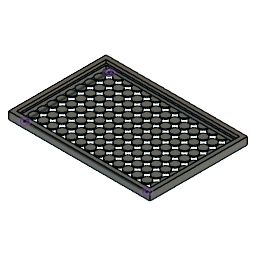
Darkfield 96 2.0 (Autodesk Fusion 360 design; units mm, degrees)
Autodesk Fusion 360 part; units mm, degrees
note: some values were not read from the file. Chosen so that the rebuilt part matches the saved one: which bodies a step acts on; which face or edge a step refers to.
sketch "Sketch1" plane through (0, 0, 0) normal (0, 0, 1) x (1, 0, 0)
  line L0 (0, 0) -> (127.6, 0)
  line L1 (127.6, 0) -> (127.6, 85.5)
  line L2 (127.6, 85.5) -> (0, 85.5)
  line L3 (0, 85.5) -> (0, 0)
  dimension "d1" = 127.6
  dimension "d2" = 85.5
  constraint horizontal L0
  constraint vertical L1
  constraint horizontal L2
  constraint vertical L3
  constraint coincident L0.start L3.end
  measures "d1" distance of L0.start L0.end
  measures "d2" distance of L0.start L2.end
ref_plane "WorkPlane1" through (0, 0, 0) normal (0, -1, 0) x (1, 0, 0)
sketch "Sketch2" plane through (0, 0, 0) normal (0, -1, 0) x (1, 0, 0)
  line L0 (0, 0) -> (0, 3)
  line L1 (0, 3) -> (-3.9, 3)
  line L2 (-3.9, 3) -> (-3.9, -4)
  line L3 (-3.9, -4) -> (1.6, -4)
  line L4 (1.6, -4) -> (1.6, 0)
  line L5 (0, 0) -> (1.6, 0)
  line L6 (-3.9, -3) -> (1.6, -3)
  line L7 (0, 0) -> (127.6, 0)
  dimension "d4" = 3
  dimension "d6" = 1
  dimension "d7" = 3
  dimension "d8" = 3.9
  dimension "d9" = 5.5
  constraint coincident L0.start L5.start
  constraint vertical L0
  constraint perpendicular L0 L1
  constraint perpendicular L1 L2
  constraint perpendicular L2 L3
  constraint perpendicular L1 L4
  constraint perpendicular L4 L5
  constraint coincident L2 L6.start
  constraint coincident L4 L6.end
  constraint perpendicular L4 L6
  measures "d4" distance of L0.start L0.end
  measures "d6" distance of L3 L6
  measures "d7" distance of L6 L7
  measures "d8" distance of L0 L2
  measures "d9" distance of L2 L4
sweep "Sweep1" add profiles "Sketch2" path "Sketch1" along L3 L0 L1 L2 section 1 makes body 1
sketch "Sketch3" plane through (0, 0, -4) normal (0, 0, 1) x (-1, 0, 0)
  line L0 (0, 0) -> (-127.6, 0)
  line L1 (-127.6, 0) -> (-127.6, -85.5)
  line L2 (-127.6, -85.5) -> (0, -85.5)
  line L3 (0, -85.5) -> (0, 0)
  line L4 (-126, -1.6) -> (-1.6, -1.6)
  line L5 (-1.6, -1.6) -> (-1.6, -83.9)
  line L6 (-1.6, -83.9) -> (-126, -83.9)
  line L7 (-126, -83.9) -> (-126, -1.6)
  circle A0 centre (-14.2, -11.3) radius 4
  line L8 (3.9, 3.9) -> (3.9, -89.4)
  line L9 (3.9, -89.4) -> (-131.5, -89.4)
  line L10 (-131.5, -89.4) -> (-131.5, 3.9)
  line L11 (-131.5, 3.9) -> (3.9, 3.9)
  line L12 (-126, -1.6) -> (-126, -83.9)
  line L13 (-126, -83.9) -> (-1.6, -83.9)
  line L14 (-1.6, -83.9) -> (-1.6, -1.6)
  line L15 (-1.6, -1.6) -> (-126, -1.6)
  dimension "d16" = 14.2
  dimension "d17" = 11.3
  dimension "d18" = 8
  measures "d16" distance of L3 A0.centre
  measures "d17" distance of L0 A0.centre
  measures "d18" diameter of A0
extrude "Extrude1" add sketch "Sketch3" along normal blind 1 separate body contours A0 makes body 2
pattern_linear "R-Pattern1" count 12 spacing 9.0182 along (1, 0, 0) count 8 spacing 8.9857 along (0, 1, 0) of bodies 2 makes body 3 at (24.2224, 11.9082, -4) makes body 4 at (34.8289, 11.8917, -4) makes body 5 at (42.2588, 11.9082, -4) makes body 6 at (52.8653, 11.8917, -4) makes body 7 at (61.8834, 11.8917, -4) makes body 8 at (70.9016, 11.8917, -4) makes body 9 at (79.9198, 11.8917, -4) makes body 10 at (88.938, 11.8917, -4) makes body 11 at (97.9562, 11.8917, -4) makes body 12 at (106.9744, 11.8917, -4) makes body 13 at (115.9925, 11.8917, -4) makes body 14 at (13.0255, 19.4085, -4) makes body 15 at (22.1898, 21.3579, -4) makes body 16 at (34.0244, 19.6188, -4) makes body 17 at (40.2262, 21.3579, -4) makes body 18 at (52.0608, 19.6188, -4) makes body 19 at (61.079, 19.6188, -4) makes body 20 at (70.0971, 19.6188, -4) makes body 21 at (79.1153, 19.6188, -4) makes body 22 at (88.1335, 19.6188, -4) makes body 23 at (97.1517, 19.6188, -4) makes body 24 at (106.1699, 19.6188, -4) makes body 25 at (115.1881, 19.6188, -4) makes body 26 at (15.3745, 28.3348, -4) makes body 27 at (24.6188, 29.8499, -4) makes body 28 at (34.2215, 28.6342, -4) makes body 29 at (42.6551, 29.8499, -4) makes body 30 at (52.2578, 28.6342, -4) makes body 31 at (61.276, 28.6342, -4) makes body 32 at (70.2942, 28.6342, -4) makes body 33 at (79.3124, 28.6342, -4) makes body 34 at (88.3306, 28.6342, -4) makes body 35 at (97.3487, 28.6342, -4) makes body 36 at (106.3669, 28.6342, -4) makes body 37 at (115.3851, 28.6342, -4) makes body 38 at (13.5921, 37.6786, -4) makes body 39 at (24.4195, 38.8357, -4) makes body 40 at (33.9068, 38.6204, -4) makes body 41 at (40.4232, 39.2996, -4) makes body 42 at (51.9432, 38.6204, -4) makes body 43 at (60.9613, 38.6204, -4) makes body 44 at (69.9795, 38.6204, -4) makes body 45 at (78.9977, 38.6204, -4) makes body 46 at (88.0159, 38.6204, -4) makes body 47 at (97.0341, 38.6204, -4) makes body 48 at (106.0522, 38.6204, -4) makes body 49 at (115.0704, 38.6204, -4) makes body 50 at (13.5921, 46.6643, -4) makes body 51 at (24.4195, 47.8214, -4) makes body 52 at (33.9068, 47.6062, -4) makes body 53 at (40.4232, 48.2853, -4) makes body 54 at (51.9432, 47.6062, -4) makes body 55 at (60.9613, 47.6062, -4) makes body 56 at (69.9795, 47.6062, -4) makes body 57 at (78.9977, 47.6062, -4) makes body 58 at (88.0159, 47.6062, -4) makes body 59 at (97.0341, 47.6062, -4) makes body 60 at (106.0522, 47.6062, -4) makes body 61 at (115.0704, 47.6062, -4) makes body 62 at (13.5921, 55.6501, -4) makes body 63 at (24.4195, 56.8071, -4) makes body 64 at (33.9068, 56.5919, -4) makes body 65 at (40.4232, 57.271, -4) makes body 66 at (51.9432, 56.5919, -4) makes body 67 at (60.9613, 56.5919, -4) makes body 68 at (69.9795, 56.5919, -4) makes body 69 at (78.9977, 56.5919, -4) makes body 70 at (88.0159, 56.5919, -4) makes body 71 at (97.0341, 56.5919, -4) makes body 72 at (106.0522, 56.5919, -4) makes body 73 at (115.0704, 56.5919, -4) makes body 74 at (16.3023, 65.3543, -4) makes body 75 at (24.8158, 65.8225, -4) makes body 76 at (34.031, 64.6358, -4) makes body 77 at (42.8522, 65.8225, -4) makes body 78 at (52.0674, 64.6358, -4) makes body 79 at (61.0856, 64.6358, -4) makes body 80 at (70.1038, 64.6358, -4) makes body 81 at (79.122, 64.6358, -4) makes body 82 at (88.1401, 64.6358, -4) makes body 83 at (97.1583, 64.6358, -4) makes body 84 at (106.1765, 64.6358, -4) makes body 85 at (115.1947, 64.6358, -4) makes body 86 at (16.3023, 74.34, -4) makes body 87 at (24.8158, 74.8082, -4) makes body 88 at (34.031, 73.6215, -4) makes body 89 at (42.8522, 74.8082, -4) makes body 90 at (52.0674, 73.6215, -4) makes body 91 at (61.0856, 73.6215, -4) makes body 92 at (70.1038, 73.6215, -4) makes body 93 at (79.122, 73.6215, -4) makes body 94 at (88.1401, 73.6215, -4) makes body 95 at (97.1583, 73.6215, -4) makes body 96 at (106.1765, 73.6215, -4) makes body 97 at (115.1947, 73.6215, -4)
sketch "Sketch4" plane through (0, 0, -3) normal (0, 0, 1) x (-1, 0, 0)
  circle A0 centre (-14.2, -74.2) radius 4
  circle A1 centre (-14.2, -65.2143) radius 4
  circle A2 centre (-23.2182, -74.2) radius 4
  dimension "d25" = 8.9857
  dimension "d26" = 9.0182
  measures "d25" distance of A0.centre A1.centre
  measures "d26" distance of A0.centre A2.centre
pattern_linear "R-Pattern2" count 2 spacing 8.9857 along (0, 1, 0) of bodies 86 87 88 89 96 97 90 95 92 91 93 94 makes body 98 at (16.3023, 83.3257, -4) makes body 99 at (24.8158, 83.7939, -4) makes body 100 at (34.031, 82.6072, -4) makes body 101 at (42.8522, 83.7939, -4) makes body 102 at (52.0674, 82.6072, -4) makes body 103 at (61.0856, 82.6072, -4) makes body 104 at (70.1038, 82.6072, -4) makes body 105 at (79.122, 82.6072, -4) makes body 106 at (88.1401, 82.6072, -4) makes body 107 at (97.1583, 82.6072, -4) makes body 108 at (106.1765, 82.6072, -4) makes body 109 at (115.1947, 82.6072, -4)
pattern_linear "R-Pattern3" count 2 spacing 9.0182 along (-1, 0, 0) of bodies 2 14 26 38 50 62 74 86 98 makes body 110 at (6.8966, 11.469, -4) makes body 111 at (4.0074, 19.4085, -4) makes body 112 at (6.3563, 28.3348, -4) makes body 113 at (4.5739, 37.6786, -4) makes body 114 at (4.5739, 46.6643, -4) makes body 115 at (4.5739, 55.6501, -4) makes body 116 at (7.2841, 65.3543, -4) makes body 117 at (7.2841, 74.34, -4) makes body 118 at (7.2841, 83.3257, -4)
ref_plane "WorkPlane2" through (63.8, 42.75, -0.5) normal (-1, 0, 0) x (0, 0, -1)
ref_plane "WorkPlane3" through (63.8, 42.75, -0.5) normal (0, -1, 0) x (0, 0, -1)
ref_plane "WorkPlane4" through (-3.9, -3.9, -4) normal (0.567406, -0.823438, 0) x (0.823438, 0.567406, 0)
mirror "Mirror1" about plane through (63.8, 42.75, -0.5) normal (0, -1, 0) of bodies 105 106 108 109 98 99 100 102 104 101 103 118 107 makes body 119 at (15.9148, 2.1453, -4) makes body 120 at (24.2224, 1.7061, -4) makes body 121 at (34.8289, 1.7226, -4) makes body 122 at (42.2588, 1.7061, -4) makes body 123 at (52.8653, 1.7226, -4) makes body 124 at (61.8834, 1.7226, -4) makes body 125 at (70.9016, 1.7226, -4) makes body 126 at (79.9198, 1.7226, -4) makes body 127 at (88.938, 1.7226, -4) makes body 128 at (97.9562, 1.7226, -4) makes body 129 at (106.9744, 1.7226, -4) makes body 130 at (115.9925, 1.7226, -4) makes body 131 at (6.8966, 2.1453, -4)
mirror "Mirror2" about plane through (63.8, 42.75, -0.5) normal (-1, 0, 0) of bodies 131 110 111 112 113 115 114 116 117 118 makes body 132 at (119.8256, 11.8917, -4) makes body 133 at (120.6301, 19.6188, -4) makes body 134 at (120.4331, 28.6342, -4) makes body 135 at (120.7478, 38.6204, -4) makes body 136 at (120.7478, 47.6062, -4) makes body 137 at (120.7478, 56.5919, -4) makes body 138 at (120.6235, 64.6358, -4) makes body 139 at (120.6235, 73.6215, -4) makes body 140 at (120.6235, 82.6072, -4) makes body 141 at (119.8256, 1.7226, -4)
sketch "Sketch5" plane through (0, 0, -4) normal (0, 0, -1) x (1, 0, 0)
  line L0 (-3.9, 3.9) -> (-3.9, -89.4)
  line L1 (-3.9, -89.4) -> (131.5, -89.4)
  line L2 (131.5, -89.4) -> (131.5, 3.9)
  line L3 (131.5, 3.9) -> (-3.9, 3.9)
  line L4 (126, -1.6) -> (126, -83.9)
  line L5 (126, -83.9) -> (1.6, -83.9)
  line L6 (1.6, -83.9) -> (1.6, -1.6)
  line L7 (1.6, -1.6) -> (126, -1.6)
  circle A0 centre (5.1818, -2.3143) radius 4
  circle A1 centre (5.1818, -83.1857) radius 4
  circle A2 centre (122.4182, -2.3143) radius 4
  line L8 (5.1818, -1.8143) -> (122.4182, -1.8143)
  line L9 (122.4182, -1.8143) -> (122.4182, -2.8143)
  line L10 (122.4182, -2.8143) -> (5.1818, -2.8143)
  line L11 (5.1818, -2.8143) -> (5.1818, -1.8143)
  line L12 (4.6818, -2.3143) -> (5.6818, -2.3143)
  line L13 (5.6818, -2.3143) -> (5.6818, -83.1857)
  line L14 (5.6818, -83.1857) -> (4.6818, -83.1857)
  line L15 (4.6818, -83.1857) -> (4.6818, -2.3143)
  dimension "d39" = 1
  dimension "d40" = 1
  dimension "d41" = 80.8714
  dimension "d42" = 117.2364
  constraint horizontal L8
  constraint vertical L9
  constraint horizontal L10
  constraint vertical L11
  constraint midpoint A0.centre L11
  constraint horizontal L12
  constraint vertical L13
  constraint horizontal L14
  constraint vertical L15
  constraint midpoint A1.centre L14
  constraint midpoint A0.centre L12
  constraint midpoint A2.centre L9
  measures "d39" distance of L8.start L10.end
  measures "d40" distance of L12.start L12.end
  measures "d41" distance of L12.start L14.end
  measures "d42" distance of L8.start L8.end
extrude "Extrude2" add sketch "Sketch5" against normal blind 1 separate body contours A0 A1 L13 L15 | A0 L10 L11 L12 L13 L15 | A1 L13 L14 L15 makes body 142
extrude "Extrude3" add sketch "Sketch5" against normal blind 1 separate body contours A0 A2 L8 L10 | A2 L8 L9 L10 | A0 L8 L10 L11 L12 L13 makes body 143
pattern_linear "R-Pattern5" count 10 spacing 8.9857 along (0, 1, 0) of bodies 143 makes body 144 at (82.0165, 11.4667, -4) makes body 145 at (82.0165, 20.4524, -4) makes body 146 at (82.0165, 29.4381, -4) makes body 147 at (82.0165, 38.4238, -4) makes body 148 at (82.0165, 47.4095, -4) makes body 149 at (82.0165, 56.3952, -4) makes body 150 at (82.0165, 65.381, -4) makes body 151 at (82.0165, 74.3667, -4) makes body 152 at (82.0165, 83.3524, -4)
pattern_linear "R-Pattern4" count 14 spacing 9.0182 along (1, 0, 0) of bodies 142 makes body 153 at (14.0333, 30.5943, -4) makes body 154 at (23.0515, 30.5943, -4) makes body 155 at (32.0697, 30.5943, -4) makes body 156 at (41.0879, 30.5943, -4) makes body 157 at (50.1061, 30.5943, -4) makes body 158 at (59.1242, 30.5943, -4) makes body 159 at (68.1424, 30.5943, -4) makes body 160 at (77.1606, 30.5943, -4) makes body 161 at (86.1788, 30.5943, -4) makes body 162 at (95.197, 30.5943, -4) makes body 163 at (104.2152, 30.5943, -4) makes body 164 at (113.2333, 30.5943, -4) makes body 165 at (122.2515, 30.5943, -4)
combine "Combine1" operation add target body 150 tool bodies 143 151 1 7 147 152 146 149 47 144 148 112 43 155 44 129 46 15 4 158 41 125 131 11 159 119 49 153 145 45 142 163 38 122 39 3 120 17 124 19 156 42 18 113 121 135 136 92 83 137 140 72 104 97 85 69 93 88 157 40 130 110 164 165 33 48 111 23 29 37 5 20 160 123 154 10 133 76 71 30 25 141 21 132 107 50 73 2 126 27 74 12 98 77 14 6 161 32 162 117 36 127 138 26 106 22 81 63 16 68 62 31 116 24 82 60 128 56 134 114 34 100 28 139 8 67 115 53 101 103 87 54 57 61 95 35 55 90 51 52 91 102 79 99 105 118 96 9 13 65 58 109 75 70 86 78 59 80 108 89 66 64 84 94
equation "d29 = -d25"
equation "d33 = -d26"
equation "d47 = -d42"
equation "d53 = d41"
